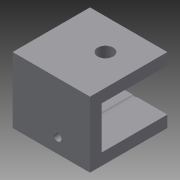
# Autodesk Inventor part: Corner2
Saved by Autodesk Inventor 2015 SP1 (Build 190203100, 203)
## iProperties
Created: 2015-08-26
Part Number: Corner2
Material: Generic
Document SubType Name: Modeling
Designer: Kartikye
Density: 1 g/cm^3
Appearance: Default
Author: Kartikye
Autodesk Inventor part; units mm, degrees
ref_plane "YZ Plane" through (0, 0, 0) normal (1, 0, 0) x (0, 1, 0)
ref_plane "XZ Plane" through (0, 0, 0) normal (0, 1, 0) x (-1, 0, 0)
ref_plane "XY Plane" through (0, 0, 0) normal (0, 0, 1) x (1, 0, 0)
sketch "Sketch1" plane through (0, 0, 0) normal (0, 1, 0) x (-1, 0, 0)
  line L0 (-5, 5) -> (5, 5)
  line L1 (5, 5) -> (5, -5)
  line L2 (5, -5) -> (-5, -5)
  line L3 (-5, -5) -> (-5, 5)
  line L4 (-5, 5) -> (5, -5) construction
  line L5 (5, 5) -> (-5, -5) construction
  point P0 (0, 0)
  dimension "d0" = 10
  dimension "d1" = 10
  constraints: 12 end point, 2 midpoint, 2 parallel, 1 horizontal, 1 perpendicular
  measures "d0" distance of L1.end L2.end
  measures "d1" distance of L0.end L1.end
extrude "Extrusion1" add sketch "Sketch1" along normal blind 1.5
sketch "Sketch2" plane through (0, 1.5, 0) normal (0, 1, 0) x (1, 0, 0)
  line L0 (-5, -5) -> (-3.5, -5)
  line L1 (-5, -5) -> (5, -5) projected
  line L2 (-3.5, -5) -> (-3.5, 3.5)
  line L3 (-3.5, 3.5) -> (5, 3.5)
  line L4 (5, 3.5) -> (5, 5)
  line L5 (5, 5) -> (-5, 5)
  line L6 (-5, 5) -> (-5, -5)
  point P0 (0, 0)
  dimension "d4" = 1.5
  dimension "d5" = 8.5
  dimension "d6" = 90
  dimension "d7" = 8.5
  dimension "d8" = 90
  dimension "d9" = 10
  dimension "d10" = 90
  constraints: 12 end point, 4 perpendicular, 1 point on line
  measures "d4" distance of L0.start L0.end
  measures "d5" distance of L0.end L2.end
  measures "d6" angle of L2 L0
  measures "d7" distance of L2.end L3.end
  measures "d8" angle of L2 L3
  measures "d9" distance of L4.end L5.end
  measures "d10" angle of L5 L4
extrude "Extrusion2" add sketch "Sketch2" along normal blind 8.5
sketch "Sketch3" plane through (0, 1.5, 0) normal (0, 1, 0) x (1, 0, 0)
  circle A0 centre (0.8, 3.1) radius 0.5
  line L0 (5, 3.5) -> (-3.5, 3.5) projected
  line L1 (-3.5, 3.5) -> (-3.5, -5) projected
  point P0 (0, 0)
  dimension "d13" = 1
  dimension "d14" = 0.4
  dimension "d15" = 4.3
  constraints: 1 centre point
  measures "d13" diameter of A0
  measures "d14" distance from line of A0.centre L0
  measures "d15" distance from line of L1 A0.centre
extrude "Extrusion3" cut sketch "Sketch3" against normal blind 8.5
sketch "Sketch4" plane through (-3.5, 1.5, -3.5) normal (0, 0, 1) x (1, 0, 0)
  circle A0 centre (1, 3.7) radius 0.5
  line L0 (8.5, 0) -> (0, 0) projected
  line L1 (0, 0) -> (0, 8.5) projected
  point P0 (3.5, -1.5)
  dimension "d18" = 1
  dimension "d19" = 3.7
  dimension "d20" = 1
  constraints: 1 centre point
  measures "d18" diameter of A0
  measures "d19" distance from line of L0 A0.centre
  measures "d20" distance from line of A0.centre L1
extrude "Extrusion4" cut sketch "Sketch4" against normal blind 8.5
sketch "Sketch5" plane through (0, 0, 0) normal (0, -1, 0) x (1, 0, 0)
  circle A0 centre (0.8, -3.1) radius 0.5
  circle A1 centre (0.8, -3.1) radius 0.5 projected
  point P0 (0, 0)
  dimension "d23" = 1
  dimension "d24" = 0
  constraints: 1 centre point
  measures "d23" diameter of A0
  measures "d24" radial gap between concentric circles of A1 A0
extrude "Extrusion5" cut sketch "Sketch5" against normal blind 10
sketch "Sketch6" plane through (-3.5, 1.5, 5) normal (1, 0, 0) x (0, 0, -1)
  circle A0 centre (4.8, 1) radius 0.5
  line L0 (0, 0) -> (8.5, 0) projected
  line L1 (8.5, 0) -> (8.5, 8.5) projected
  point P0 (5, -1.5)
  dimension "d27" = 1
  dimension "d28" = 1
  dimension "d29" = 3.7
  constraints: 1 centre point
  measures "d27" diameter of A0
  measures "d28" distance from line of L0 A0.centre
  measures "d29" distance from line of L1 A0.centre
extrude "Extrusion6" cut sketch "Sketch6" against normal blind 2
sketch "Sketch7" plane through (-5, 0, 5) normal (0, 0, 1) x (1, 0, 0)
  line L0 (0, 0) -> (10, 0)
  line L1 (10, 0) -> (10, 10)
  line L2 (10, 10) -> (0, 10)
  line L3 (0, 10) -> (0, 0)
  point P0 (5, 0)
  constraints: 8 end point, 2 parallel, 1 horizontal, 1 perpendicular
extrude "Extrusion7" cut sketch "Sketch7" against normal blind 3
sketch "Sketch8" plane through (-5, 0, 2) normal (0, 0, 1) x (1, 0, 0)
  line L0 (0, 0) -> (10, 0)
  line L1 (10, 0) -> (10, 10)
  line L2 (10, 10) -> (0, 10)
  line L3 (0, 10) -> (0, 0)
  point P0 (5, 0)
  constraints: 8 end point, 2 parallel, 1 horizontal, 1 perpendicular
extrude "Extrusion8" add sketch "Sketch8" along normal blind 1.5
sketch "Sketch9" plane through (-5, 0, 3.5) normal (0, 0, 1) x (1, 0, 0)
  circle A0 centre (6, 6) radius 1
  line L0 (0, 0) -> (10, 0) projected
  line L1 (0, 10) -> (0, 0) projected
  point P0 (5, 0)
  dimension "d36" = 2
  dimension "d37" = 6
  dimension "d38" = 6
  constraints: 1 centre point
  measures "d36" diameter of A0
  measures "d37" distance from line of A0.centre L0
  measures "d38" distance from line of L1 A0.centre
extrude "Extrusion9" cut sketch "Sketch9" against normal blind 1.5
body "Solid1"
